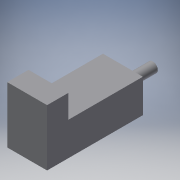
# Autodesk Inventor part: motor
Saved by Autodesk Inventor 2018 (Build 220112000, 112)
## iProperties
Created: 2016-02-02
Part Number: motor
Material: Générique
Document SubType Name: Modeling
Designer: Gregwar
Density: 1 g/cm^3
Appearance: Par défaut
d0: 10,000 mm
d1: 12,000 mm
d2: 22,400 mm
d3: 0,00 deg
d4: 3,000 mm
d5: 9,000 mm
d6: 0,00 deg
d7: 17,000 mm
d8: 6,400 mm
d9: 0,00 deg
motor_width: 12,000 mm
motor_height: 10,000 mm
Author: Gregwar
Autodesk Inventor part; units mm, degrees
ref_plane "YZ Plane" through (0, 0, 0) normal (1, 0, 0) x (0, 1, 0)
ref_plane "XZ Plane" through (0, 0, 0) normal (0, 1, 0) x (-1, 0, 0)
ref_plane "XY Plane" through (0, 0, 0) normal (0, 0, 1) x (1, 0, 0)
sketch "Esquisse1" plane through (0, 0, 0) normal (0, 1, 0) x (-1, 0, 0)
  line L0 (0, 0) -> (12, 0)
  line L1 (12, 0) -> (12, -10)
  line L2 (12, -10) -> (0, -10)
  line L3 (0, -10) -> (0, 0)
  dimension "motor_height" = 10
  dimension "motor_width" = 12
  constraints: 8 end point, 2 parallel, 1 horizontal, 1 perpendicular
  measures "motor_height" distance of L2.end L0.start
  measures "motor_width" distance of L0.start L0.end
extrude "Extrusion1" add sketch "Esquisse1" along normal blind 22.4
sketch "Esquisse2" plane through (0, 22.4, 0) normal (0, 1, 0) x (1, 0, 0)
  line L0 (-12, 0) -> (0, 0) construction
  line L1 (0, 0) -> (0, 10) construction
  line L2 (0, 10) -> (-12, 10) construction
  line L3 (-12, 10) -> (-12, 0) construction
  line L4 (-12, 5) -> (0, 5) construction
  line L5 (0, 0) -> (0, 10) construction
  circle A0 centre (-6, 5) radius 1.5
  dimension "d4" = 3
  constraints: 3 midpoint, 2 end point, 1 centre point
  measures "d4" diameter of A0
extrude "Extrusion2" add sketch "Esquisse2" along normal blind 9
sketch "Esquisse3" plane through (0, 0, 0) normal (0, -1, 0) x (1, 0, 0)
  line L0 (0, 0) -> (-12, 0) construction
  line L1 (-12, 0) -> (-12, -10) construction
  line L2 (-12, -10) -> (0, -10) construction
  line L3 (0, -10) -> (0, 0) construction
  line L4 (0, -10) -> (-12, -10)
  line L5 (-12, -10) -> (-12, 7)
  line L6 (-12, 7) -> (0, 7)
  line L7 (0, 7) -> (0, -10)
  line L8 (-12, 0) -> (-12, -10) projected
  dimension "d7" = 17
  constraints: 8 end point, 2 parallel, 1 collinear, 1 horizontal, 1 perpendicular
  measures "d7" distance between parallel lines of L2 L6
extrude "Extrusion3" add sketch "Esquisse3" along normal blind 6.4
